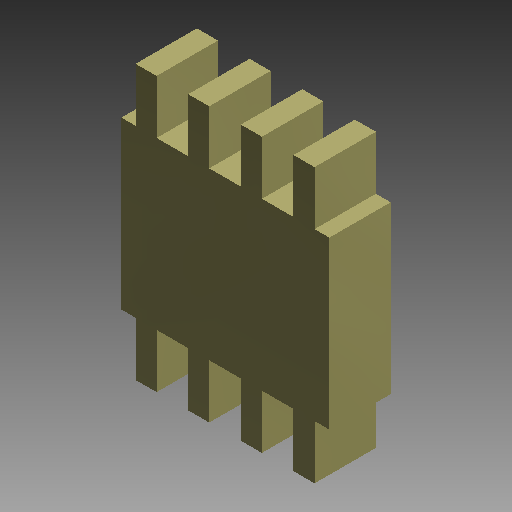
# Autodesk Inventor part: NCV8402AD
Saved by Autodesk Inventor 2018.2 (Build 222227000, 227)
## iProperties
Part Number: NCV8402AD
Material: Generic
Document SubType Name: Modeling
Designer: autocad
Appearance: NCV8402AD-SOIC8, NCV8402AD
Author: autocad
Autodesk Inventor part; units mm, degrees
ref_plane "YZ Plane" through (0, 0, 0) normal (1, 0, 0) x (0, 1, 0)
ref_plane "XZ Plane" through (0, 0, 0) normal (0, 1, 0) x (-1, 0, 0)
ref_plane "XY Plane" through (0, 0, 0) normal (0, 0, 1) x (1, 0, 0)
sketch "NCV8402AD-SOIC8, NCV8402AD_162" plane through (0, 0, 0) normal (0, 0, 1) x (1, 0, 0)
  line L0 (-2.159, 2.0066) -> (-2.159, 3.302)
  line L1 (-2.159, 3.302) -> (-1.651, 3.302)
  line L2 (-1.651, 3.302) -> (-1.651, 2.0066)
  line L3 (-1.651, 2.0066) -> (-0.889, 2.0066)
  line L4 (-0.889, 2.0066) -> (-0.889, 3.302)
  line L5 (-0.889, 3.302) -> (-0.381, 3.302)
  line L6 (-0.381, 3.302) -> (-0.381, 2.0066)
  line L7 (-0.381, 2.0066) -> (0.381, 2.0066)
  line L8 (0.381, 2.0066) -> (0.381, 3.302)
  line L9 (0.381, 3.302) -> (0.889, 3.302)
  line L10 (0.889, 3.302) -> (0.889, 2.0066)
  line L11 (0.889, 2.0066) -> (1.651, 2.0066)
  line L12 (1.651, 2.0066) -> (1.651, 3.302)
  line L13 (1.651, 3.302) -> (2.159, 3.302)
  line L14 (2.159, 3.302) -> (2.159, 2.0066)
  line L15 (2.159, 2.0066) -> (2.5146, 2.0066)
  line L16 (2.5146, 2.0066) -> (2.5146, -2.0016)
  line L17 (2.5146, -2.0016) -> (2.159, -2.0016)
  line L18 (2.159, -2.0016) -> (2.159, -3.302)
  line L19 (2.159, -3.302) -> (1.651, -3.302)
  line L20 (1.651, -3.302) -> (1.651, -2.0016)
  line L21 (1.651, -2.0016) -> (0.889, -2.0016)
  line L22 (0.889, -2.0016) -> (0.889, -3.302)
  line L23 (0.889, -3.302) -> (0.381, -3.302)
  line L24 (0.381, -3.302) -> (0.381, -2.0016)
  line L25 (0.381, -2.0016) -> (-0.381, -2.0016)
  line L26 (-0.381, -2.0016) -> (-0.381, -3.302)
  line L27 (-0.381, -3.302) -> (-0.889, -3.302)
  line L28 (-0.889, -3.302) -> (-0.889, -2.0016)
  line L29 (-0.889, -2.0016) -> (-1.651, -2.0016)
  line L30 (-1.651, -2.0016) -> (-1.651, -3.302)
  line L31 (-1.651, -3.302) -> (-2.159, -3.302)
  line L32 (-2.159, -3.302) -> (-2.159, -2.0016)
  line L33 (-2.159, -2.0016) -> (-2.5016, -2.0016)
  line L34 (-2.5016, -2.0016) -> (-2.5016, 2.0066)
  line L35 (-2.5016, 2.0066) -> (-2.159, 2.0066)
  constraints: 72 end point
extrude "Extrusion1" add sketch "NCV8402AD-SOIC8, NCV8402AD_162" along normal blind 1.48
body "Solid1"
